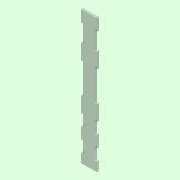
# Autodesk Inventor part: Right_wall
Saved by Autodesk Inventor 2015 (Build 190159000, 159)
## iProperties
Created: 2015-06-19
Part Number: Right_wall
Material: Generic
Document SubType Name: Modeling
Designer: Openlab
Density: 1 g/cm^3
Appearance: Polycarbonate - Clear
Author: Openlab
Autodesk Inventor part; units mm, degrees
ref_plane "YZ Plane" through (0, 0, 0) normal (1, 0, 0) x (0, 1, 0)
ref_plane "XZ Plane" through (0, 0, 0) normal (0, 1, 0) x (-1, 0, 0)
ref_plane "XY Plane" through (0, 0, 0) normal (0, 0, 1) x (1, 0, 0)
sketch "Sketch1" plane through (0, 0, 0) normal (0, 1, 0) x (-1, 0, 0)
  line L0 (21, -15) -> (18.25, -15)
  line L1 (21, -38) -> (18.25, -38)
  line L2 (21, -133) -> (18.25, -133)
  line L3 (21, -58) -> (18.25, -58)
  line L4 (21, -118) -> (18.25, -118)
  line L5 (21, -98) -> (18.25, -98)
  line L6 (2.75, -58) -> (0, -58)
  line L7 (2.75, -98) -> (0, -98)
  line L8 (2.75, -118) -> (0, -118)
  line L9 (2.75, -133) -> (0, -133)
  line L10 (2.75, -38) -> (0, -38)
  line L11 (2.75, -15) -> (0, -15)
  line L12 (21, -148) -> (21, -133)
  line L13 (21, -118) -> (21, -98)
  line L14 (21, -58) -> (21, -38)
  line L15 (21, -15) -> (21, 0)
  line L16 (0, -148) -> (0, -133)
  line L17 (0, -118) -> (0, -98)
  line L18 (0, -58) -> (0, -38)
  line L19 (0, -15) -> (0, 0)
  line L20 (18.25, -133) -> (18.25, -118)
  line L21 (18.25, -98) -> (18.25, -58)
  line L22 (18.25, -38) -> (18.25, -15)
  line L23 (2.75, -133) -> (2.75, -118)
  line L24 (2.75, -98) -> (2.75, -58)
  line L25 (2.75, -38) -> (2.75, -15)
  line L26 (21, -58) -> (21, -38) construction
  line L27 (21, 0) -> (0, 0)
  line L28 (10.5, -68) -> (10.5, -97) construction
  line L29 (18.25, -148) -> (18.25, -163)
  line L30 (18.25, -163) -> (21, -163)
  line L31 (21, -163) -> (21, -175)
  line L32 (21, -175) -> (0, -175)
  line L33 (0, -175) -> (0, -163)
  line L34 (0, -163) -> (2.75, -163)
  line L35 (2.75, -148) -> (2.75, -163)
  line L36 (21, -148) -> (18.25, -148)
  line L37 (2.75, -148) -> (0, -148)
  dimension "d7" = 23
  dimension "d8" = 20
  dimension "d9" = 40
  dimension "d10" = 20
  dimension "d11" = 15
  dimension "d28" = 15.5
  dimension "d31" = 2.75
  dimension "d42" = 15
  dimension "d44" = 12
  dimension "d45" = 15
  dimension "d47" = 15
  constraints: 77 end point, 29 collinear, 10 perpendicular, 4 vertical, 2 parallel, 2 point on line, 1 other
  measures "d7" distance between parallel lines of L1 L0
  measures "d8" distance between parallel lines of L3 L1
  measures "d9" distance between parallel lines of L5 L3
  measures "d10" distance between parallel lines of L4 L5
  measures "d11" distance between parallel lines of L2 L4
  measures "d28" distance between parallel lines of L23 L20
  measures "d31" distance between parallel lines of L22 L15
  measures "d42" distance from line of L0.start L27
  measures "d44" distance of L30.end L31.end
  measures "d45" distance of L29.start L29.end
  measures "d47" distance of L12.start L2.start
extrude "Extrusion3" add sketch "Sketch1" along normal blind 3
body "Solid3"
